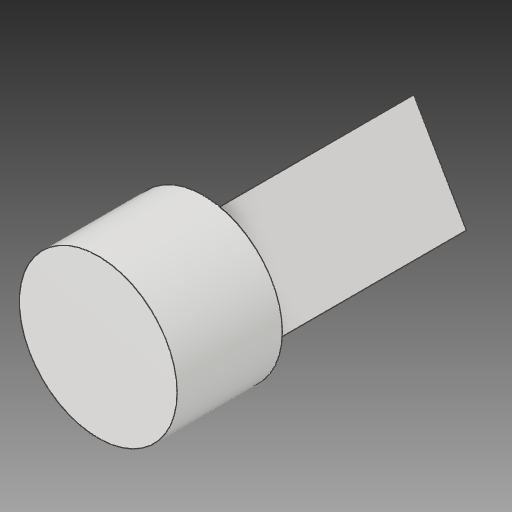
# Autodesk Inventor part: Driver Shaft
Saved by Autodesk Inventor 2018 (Build 220112000, 112)
## iProperties
Created: 2018-01-20
Part Number: Driver Shaft
Material: ABS Plastic
Document SubType Name: Modeling
Designer: Rus
Density: 1.06 g/cm^3
Appearance: Smooth - White
Mass: 1.69403 g
Surface Area: 10.2127 cm^2
Volume: 1.59815 cm^3
Author: Rus
Autodesk Inventor part; units mm, degrees
ref_plane "YZ Plane" through (0, 0, 0) normal (1, 0, 0) x (0, 1, 0)
ref_plane "XZ Plane" through (0, 0, 0) normal (0, 1, 0) x (-1, 0, 0)
ref_plane "XY Plane" through (0, 0, 0) normal (0, 0, 1) x (1, 0, 0)
sketch "Sketch1" plane through (0, 0, 0) normal (0, 0, 1) x (1, 0, 0)
  line L0 (0, 10.9985) -> (9.525, -5.4993)
  line L1 (9.525, -5.4993) -> (-9.525, -5.4993)
  line L2 (-9.525, -5.4993) -> (0, 10.9985)
  line L3 (-4.2333, -2.4441) -> (0, 4.8882)
  line L4 (0, 4.8882) -> (4.2333, -2.4441)
  line L5 (4.2333, -2.4441) -> (-4.2333, -2.4441)
  point P0 (0, 0)
  point P1 (0, 0)
  point P2 (0, 0)
  dimension "d0" = 19.05
  dimension "d1" = 8.4667
  constraints: 12 end point, 2 coincident, 2 horizontal, 14 other
  measures "d0" distance of L0.end L1.end
  measures "d1" distance of L4.end L3.start
extrude "Extrusion1" add sketch "Sketch1" against normal blind 16.9333 contours L3 L4 L5
sketch "Sketch2" plane through (0, 0, 0) normal (0, 0, 1) x (1, 0, 0)
  circle A0 centre (0, 0) radius 6.35
  dimension "d4" = 12.7
  constraints: 1 centre point, 1 coincident
  measures "d4" diameter of A0
extrude "Extrusion2" add sketch "Sketch2" along normal blind 8.4667
body "Solid1"
